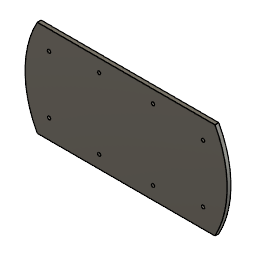
FEKTBOT_RPlidar_ver_1_2 (Autodesk Fusion 360 design; units mm, degrees)
part number: 2026-09-01-10-12-56-077
Autodesk Fusion 360 part; units mm, degrees
sketch "Sketch1" plane through (0, 0, 0) normal (0, 0, 1) x (1, 0, 0)
  circle A0 centre (-80, -30) radius 1.65
  line L0 (0, 2.5) -> (0, 20)
  line L1 (20, 0) -> (2.5, 0)
  circle A1 centre (-80, 30) radius 1.65
  circle A2 centre (80, -30) radius 1.65
  circle A3 centre (80, 30) radius 1.65
  line L2 (-28, 36.75) -> (28, 36.75) construction
  line L3 (28, 36.75) -> (28, -36.75) construction
  line L4 (28, -36.75) -> (-28, -36.75) construction
  line L5 (-28, -36.75) -> (-28, 36.75) construction
  circle A4 centre (-28, 36.75) radius 1.6
  circle A5 centre (28, 36.75) radius 1.6
  circle A6 centre (-28, -36.75) radius 1.6
  circle A7 centre (28, -36.75) radius 1.6
  line L6 (-92.3309, -50) -> (92.3309, -50)
  line L7 (-92.3309, 50) -> (92.3309, 50)
  arc A8 (-92.3309, 50) -> (-92.3309, -50) centre (0, 0) ccw
  arc A9 (92.3309, -50) -> (92.3309, 50) centre (0, 0) ccw
  dimension "d1" = 210
  dimension "d2" = 3.3
  dimension "d3" = 80
  dimension "d4" = 30
  dimension "d5" = 56
  dimension "d6" = 73.5
  dimension "d7" = 3.2
  dimension "d8" = 3.2
  dimension "d9" = 3.2
  dimension "d10" = 3.2
  dimension "d11" = 50
  constraint coincident A8.centre A9.centre
  constraint symmetric A0 L1 A1
  constraint symmetric A0 L0 A2
  constraint symmetric L0 A1 A3
  constraint horizontal L2
  constraint vertical L3
  constraint horizontal L4
  constraint vertical L5
  constraint symmetric L0 L3 L5
  constraint symmetric L1 L2 L4
  constraint coincident L2.start L5.end
  constraint coincident L2.end L3.start
  constraint coincident L4.end L5.start
  constraint coincident L3.end L4.start
  constraint horizontal L6
  constraint concentric A8 A9
  measures "d1" diameter of A8
  measures "d2" diameter of A0
  measures "d3" distance of A0.centre L0
  measures "d4" distance of A0.centre L1
  measures "d5" distance of L2.start L2.end
  measures "d6" distance of L2.start L4.end
  measures "d7" diameter of A4
  measures "d8" diameter of A5
  measures "d9" diameter of A6
  measures "d10" diameter of A7
  measures "d11" distance of L1 L6
extrude "Extrude1" add sketch "Sketch1" along normal blind 4
equation "d6 = 28 mm + 45.5 mm"
